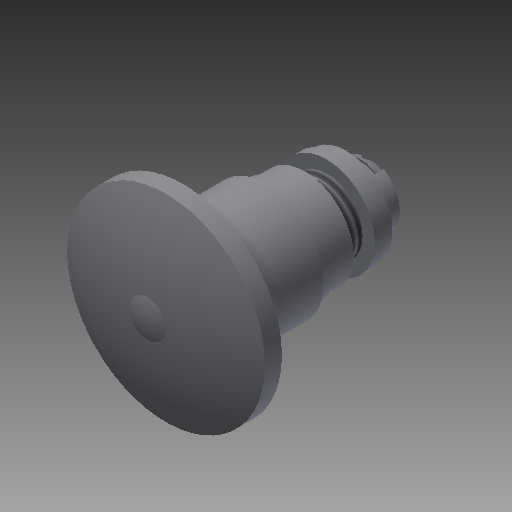
# Autodesk Inventor part: 152861
Saved by Autodesk Inventor 2019.3 (Build 233278000, 278)
## iProperties
Category: PARTsolutions
Company: MOELLER
Created: 2018-10-25
Part Number: 152861
Material: Generic
Catalog Web Link: www.cadenas.de
Description: Stop/halt pushbutton, IP67, IP69K-
Vendor: MOELLER
Document SubType Name: Modeling
Designer: psadmin
Manufacturer: MOELLER
Mass: 67.8113 g
Surface Area: 122.665 cm^2
Volume: 67.8113 cm^3
Density: 1 g/cm^3
Appearance: PSOLRGB-175-175-175
PSOL_IDENT_0: {$CADENAS_DATA\23d-libs\moeller\2\4\6\8\40\43.prj},192 {VTYP=3D},{NB=152861},{LINA=152861},{NN=Stop/
PSOL_IDENT_1: halt pushbutton, IP67, IP69K},{DATE=04.10.2018 12:16:42},{GEOMDATE=04.10.2018 08:29:25},{VERSION=v18
PSOL_IDENT_2: 1004082925},{LINEID=60},{WBVAR=},{WBNUMERIC=}  {NB=152861},{LINA=152861},{KT=DUMMY},{PFOTO=1160pic-1
PSOL_IDENT_3: 071.jpg},{PLID=152861},{DATA_SHEET=Data sheet},{MANUTYPEDESC=M22-PVL60P},{DESCSHORT=Emergency-stop/o
PSOL_IDENT_4: ff pushbutton, D=60mm, illuminated, pull release},{DESCLONG=Emergency stop/emergency switching off p
PSOL_IDENT_5: ushbutton, Product range: RMQ-Titan, Single unit, Design: Palm-tree shape, Diameter: 60 mm, Illumina
PSOL_IDENT_6: tion: Illuminated with LED element, Pull-to-release function, Description: Tamper-proof according to
PSOL_IDENT_7: ISO 13850/EN 418, Colour Mushroom head: Red, Colour Base: yellow, Degree of Protection: IP67, IP69K
PSOL_IDENT_8: , Connection to SmartWire-DT: no, Instructions: Max. number of contacts: four M22-(C)K01, …10 or two
PSOL_IDENT_9: M22-(C)K02, …20, …11, Standards: IEC/EN 60947, VDE 0660},{EAN=4015081496396},{ECLASS_8_1=27-37-12-1
PSOL_IDENT_10: 2},{PACKAGED_WEIGHT=0.051},{DATA_SHEET_=http://datasheet.moeller.net/datasheet.php?model=152861&loca
PSOL_IDENT_11: le=en_GB},{DATA_SHEET_ENG=http://datasheet.moeller.net/datasheet.php?model=152861&locale=en_GB},{DAT
PSOL_IDENT_12: A_SHEET_DEU=http://datasheet.moeller.net/datasheet.php?model=152861&locale=de_DE}
NN: Stop/halt pushbutton, IP67, IP69K
NB: 152861
NBSYN: $PLID.
LINA: 152861
PFOTO: 1160pic-1071.jpg
PLID: 152861
DATA_SHEET: Data sheet
MANUTYPEDESC: M22-PVL60P
DESCSHORT: Emergency-stop/off pushbutton, D=60mm, illuminated, pull release
DESCLONG: Emergency stop/emergency switching off pushbutton, Product range: RMQ-Titan, Single unit, Design: Palm-tree shape, Diameter: 60 mm, Illumination: Illuminated with LED element, Pull-to-release function, Description: Tamper-proof according to ISO 13850/EN 418, Colour Mushroom head: Red, Colour Base: yellow, Degree of Protection: IP67, IP69K, Connection to SmartWire-DT: no, Instructions: Max. number of contacts: four M22-(C)K01, …10 or two M22-(C)K02, …20, …11, Standards: IEC/EN 60947, VDE 0660
EAN: 4015081496396
ECLASS_8_1: 27-37-12-12
PACKAGED_WEIGHT: 0.051
SUPPLIER: MOELLER
ARTICLENO: 152861
BOMINFO: 152861
CREATOR: CADENAS GmbH
Title: 152861
Author: Cadenas PARTsolutions
Autodesk Inventor part; units mm, degrees
ref_plane "YZ Plane" through (0, 0, 0) normal (1, 0, 0) x (0, 1, 0)
ref_plane "XZ Plane" through (0, 0, 0) normal (0, 1, 0) x (-1, 0, 0)
ref_plane "XY Plane" through (0, 0, 0) normal (0, 0, 1) x (1, 0, 0)
sketch "Sketch_1" plane through (0, 0, 0) normal (0, 1, 0) x (-1, 0, 0)
  line L0 (0, 66.6946) -> (0, 0)
  line L1 (0, 0) -> (-10, 0)
  line L2 (-10, 0) -> (-10, 18.3073)
  line L3 (-10, 18.3073) -> (-14, 18.3073)
  line L4 (-14, 18.3073) -> (-14, 18.8)
  line L5 (-14, 18.8) -> (-14.8, 18.8)
  line L6 (-14.8, 18.8) -> (-14.8, 25.1)
  line L7 (-14.8, 25.1) -> (-15.4, 25.1)
  line L8 (-15.4, 25.1) -> (-15.4, 30.7005)
  line L9 (-15.4, 30.7005) -> (-17.55, 30.7005)
  line L10 (-17.55, 30.7005) -> (-17.55, 43.8132)
  arc A0 (-17.55, 43.8132) -> (-28.8609, 55.7934) centre (-29.55, 43.8132) ccw
  line L11 (-28.8609, 55.7934) -> (-30, 55.7934)
  line L12 (-30, 55.7934) -> (-30, 60.9342)
  arc A1 (-5.6001, 66.5008) -> (-30, 60.9342) centre (0, -14.3054) ccw
  arc A2 (0, 67.3008) -> (-5.6001, 66.5008) centre (0, 47.3008) ccw
  line L13 (0, 67.3008) -> (0, 0)
  constraints: 28 end point, 6 point on circle, 3 centre point
revolve "Revolution1" add sketch "Sketch_1" angle 360 about axis through (0, 0, 66.6946) along (0, 0, 1)
sketch "Sketch_9" plane through (0, 0, 0) normal (0, 1, 0) x (-1, 0, 0)
  line L0 (0, 18.3073) -> (0, 6.55)
  line L1 (0, 6.55) -> (-9.4665, 6.55)
  line L2 (-9.4665, 6.55) -> (-11, 8.0835)
  line L3 (-11, 8.0835) -> (-11, 18.3073)
  line L4 (-11, 18.3073) -> (0, 18.3073)
  line L5 (0, 18.3073) -> (0, 6.55)
  constraints: 12 end point
revolve "Revolution2" add sketch "Sketch_9" angle 360 about axis through (0, 0, 18.3073) along (0, 0, 1)
thread "Thread1" size "M22x2.5" class "6g" standard "ISO Metric profile" length 8.6304
sketch "Sketch_2" plane through (0, 0, 0) normal (1, 0, 0) x (0, 1, 0)
  line L0 (0, 6.3073) -> (0, 12.3073)
  line L1 (11, 12.3073) -> (10.188, 11.4953)
  line L2 (10.188, 11.4953) -> (10.188, 7.1193)
  line L3 (10.188, 7.1193) -> (11, 6.3073)
  line L4 (11, 6.3073) -> (14, 6.3073)
  line L5 (14, 6.3073) -> (14, 9.3073)
  line L6 (14, 9.3073) -> (14.75, 9.3073)
  line L7 (14.75, 9.3073) -> (14.75, 12.3073)
  line L8 (14.75, 12.3073) -> (11, 12.3073)
  constraints: 18 end point
sketch "Sketch_5" plane through (0, 0, 0) normal (1, 0, 0) x (0, 1, 0)
  line L0 (16.375, 6.55) -> (7, 6.55)
  line L1 (7, 6.55) -> (7, 0)
  line L2 (7, 0) -> (16.375, 0)
  line L3 (16.375, 0) -> (16.375, 6.55)
  constraints: 8 end point
extrude "Extrusion1" cut sketch "Sketch_5" along normal mid plane 10.2
sketch "Sketch_7" plane through (0, 0, 0) normal (1, 0, 0) x (0, 1, 0)
  line L0 (-7, 6.55) -> (-16.375, 6.55)
  line L1 (-16.375, 6.55) -> (-16.375, 0)
  line L2 (-16.375, 0) -> (-7, 0)
  line L3 (-7, 0) -> (-7, 6.55)
  constraints: 8 end point
extrude "Extrusion2" cut sketch "Sketch_7" along normal mid plane 10.2
sketch "Sketch_6" plane through (0, 0, 0) normal (1, 0, 0) x (0, 1, 0)
  line L0 (0, 0) -> (0, 6.55)
  line L1 (10.05, 6.55) -> (5, 6.55)
  line L2 (5, 6.55) -> (5, 0)
  line L3 (5, 0) -> (9, 0)
  line L4 (9, 0) -> (10, 2.15)
  line L5 (10, 2.15) -> (10, 2.3)
  line L6 (10, 2.3) -> (9.25, 2.3)
  line L7 (9.25, 2.3) -> (9.05, 2.5)
  line L8 (9.05, 2.5) -> (9.05, 5.55)
  line L9 (9.05, 5.55) -> (10.05, 6.55)
  constraints: 20 end point
revolve "Revolution3" add sketch "Sketch_6" angle 360 about axis through (0, 0, 0) along (0, 0, -1)
sketch "Sketch_4" plane through (0, 0, 0) normal (0, 1, 0) x (-1, 0, 0)
  line L0 (2.1213, -0.6213) -> (0, 1.5)
  line L1 (0, 1.5) -> (-2.1213, -0.6213)
  line L2 (-2.1213, -0.6213) -> (0, -2.7426)
  line L3 (0, -2.7426) -> (2.1213, -0.6213)
  constraints: 8 end point
extrude "Extrusion3" cut sketch "Sketch_4" along normal blind 10
sketch "Sketch_8" plane through (0, 0, 16.3) normal (0, 0, 1) x (1, 0, 0)
  line L0 (-1.5, 7.2) -> (1.5, 7.2)
  line L1 (1.5, 7.2) -> (1.5, 12.2)
  line L2 (1.5, 12.2) -> (-1.5, 12.2)
  line L3 (-1.5, 12.2) -> (-1.5, 7.2)
  constraints: 8 end point
extrude "Extrusion4" add sketch "Sketch_8" along normal blind 3
revolve "Revolution4" add sketch "Sketch_2" angle 360 about axis through (0, 0, 6.3073) along (0, 0, -1)
thread "Thread2" size "M22x1.5" class "6H" standard "ISO Metric profile" length 4.376
body "Solid1"
